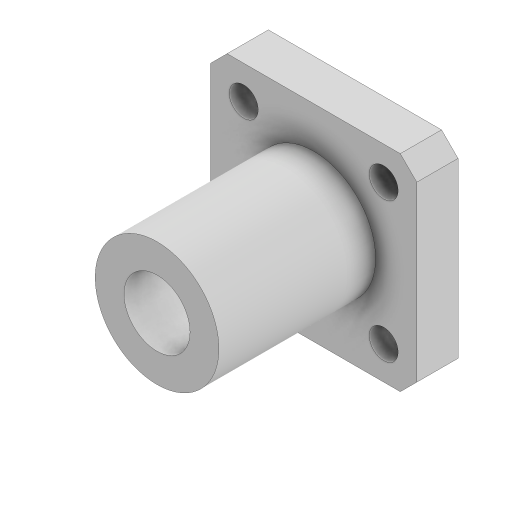
# Autodesk Inventor part: RODAMIENTO LINEAL
Saved by Autodesk Inventor 2024 (Build 280153000, 153)
## iProperties
Created: 2024-06-26
Part Number: RODAMIENTO LINEAL
Material: Generic
Document SubType Name: Modeling
Designer: Jhuliams
Density: 1 g/cm^3
Appearance: Default
Author: Jhuliams
Autodesk Inventor part; units mm, degrees
ref_plane "YZ Plane" through (0, 0, 0) normal (1, 0, 0) x (0, 1, 0)
ref_plane "XZ Plane" through (0, 0, 0) normal (0, 1, 0) x (-1, 0, 0)
ref_plane "XY Plane" through (0, 0, 0) normal (0, 0, 1) x (1, 0, 0)
sketch "Sketch1" plane through (0, 0, 0) normal (0, 0, 1) x (1, 0, 0)
  line L0 (-12.5, 12.5) -> (12.5, 12.5)
  line L1 (12.5, 12.5) -> (12.5, -12.5)
  line L2 (12.5, -12.5) -> (-12.5, -12.5)
  line L3 (-12.5, -12.5) -> (-12.5, 12.5)
  line L4 (-12.5, 12.5) -> (12.5, -12.5) construction
  line L5 (12.5, 12.5) -> (-12.5, -12.5) construction
  point P0 (0, 0)
  dimension "d0" = 25
  dimension "d1" = 25
  constraints: 12 end point, 2 midpoint, 2 parallel, 1 horizontal, 1 perpendicular
  measures "d0" distance of L1.end L2.end
  measures "d1" distance of L0.end L1.end
extrude "Extrusion1" add sketch "Sketch1" along normal blind 5
sketch "Sketch2" plane through (0, 0, 5) normal (0, 0, 1) x (1, 0, 0)
  circle A0 centre (0, 0) radius 7.5
  dimension "d4" = 15
  constraints: 1 centre point, 1 coincident
  measures "d4" diameter of A0
extrude "Extrusion2" add sketch "Sketch2" along normal blind 19
sketch "Sketch3" plane through (0, 0, 24) normal (0, 0, 1) x (1, 0, 0)
  circle A0 centre (0, 0) radius 4
  dimension "d7" = 8
  constraints: 1 centre point, 1 coincident
  measures "d7" diameter of A0
extrude "Extrusion3" cut sketch "Sketch3" against normal blind 30
sketch "Sketch4" plane through (0, 0, 0) normal (0, 0, -1) x (-1, 0, 0)
  circle A0 centre (0, 0) radius 12
  line L0 (-12.5, -12.5) -> (-12.5, 12.5) projected
  line L1 (12.5, 12.5) -> (12.5, -12.5) projected
  line L2 (-12.5, 12.5) -> (8.4853, -8.4853)
  circle A1 centre (8.4853, -8.4853) radius 1.75
  circle A2 centre (8.4853, 8.4853) radius 1.75
  circle A3 centre (-8.4853, 8.4853) radius 1.75
  circle A4 centre (-8.4853, -8.4853) radius 1.75
  dimension "d10" = 24
  dimension "d11" = 3.5
  dimension "d14" = 360
  constraints: 4 centre point, 2 coincident, 2 end point, 12 other
  measures "d11" diameter of A1
extrude "Extrusion4" cut sketch "Sketch4" against normal blind 30 contours A2 A0 | A0 A2 | A1 A0 | A0 L2 A1 | A0 A1 L2 | A3 L2 A0 | A0 L2 A3 | A3 A0 L2 | A0 A3 L2 | A4 A0 | A0 A4
chamfer "Chamfer1" distance 2 angle 45 4 edges at (12.5, 12.5, 2.5) (-12.5, 12.5, 2.5) (-12.5, -12.5, 2.5) (12.5, -12.5, 2.5)
body "Solid1"
